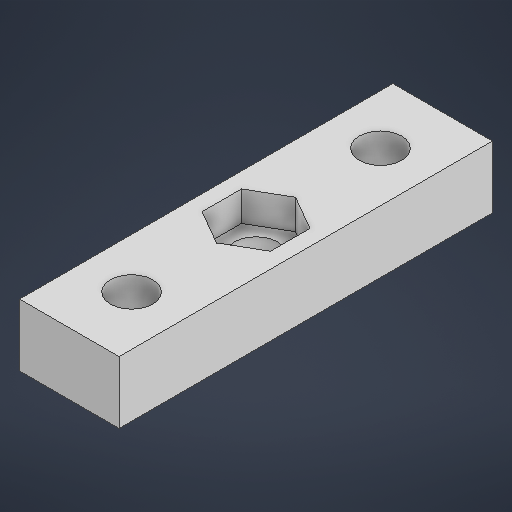
# Autodesk Inventor part: turning clip bottom
Saved by Autodesk Inventor 2025.2 (Build 292293000, 293)
## iProperties
Created: 2025-05-25
Part Number: turning clip bottom
Material: Generic
Document SubType Name: Modeling
Designer: klawy
Density: 1 g/cm^3
Appearance: Default
Author: klawy
Autodesk Inventor part; units mm, degrees
ref_plane "YZ Plane" through (0, 0, 0) normal (1, 0, 0) x (0, 1, 0)
ref_plane "XZ Plane" through (0, 0, 0) normal (0, 1, 0) x (-1, 0, 0)
ref_plane "XY Plane" through (0, 0, 0) normal (0, 0, 1) x (1, 0, 0)
sketch "Sketch1" plane through (0, 0, 0) normal (0, 1, 0) x (-1, 0, 0)
  line L0 (-4, -15) -> (4, -15)
  line L1 (4, -15) -> (4, 15)
  line L2 (4, 15) -> (-4, 15)
  line L3 (-4, 15) -> (-4, -15)
  line L4 (-4, -15) -> (4, 15) construction
  line L5 (4, -15) -> (-4, 15) construction
  circle A0 centre (0, 0) radius 1.75
  dimension "d0" = 8
  dimension "d1" = 30
  dimension "d2" = 3.5
  constraints: 12 end point, 2 midpoint, 2 parallel, 1 centre point, 1 coincident, 1 horizontal, 1 perpendicular
  measures "d0" distance of L1.end L2.end
  measures "d1" distance of L0.end L1.end
  measures "d2" diameter of A0
extrude "Extrusion1" add sketch "Sketch1" along normal blind 5
sketch "Sketch2" plane through (0, 5, 0) normal (0, 1, 0) x (1, 0, 0)
  circle A0 centre (0, 0) radius 1.75 projected
  circle A1 centre (0, 0) radius 2.75 construction
  line L0 (-2.75, 1.5877) -> (0, 3.1754)
  line L1 (0, 3.1754) -> (2.75, 1.5877)
  line L2 (2.75, 1.5877) -> (2.75, -1.5877)
  line L3 (2.75, -1.5877) -> (0, -3.1754)
  line L4 (0, -3.1754) -> (-2.75, -1.5877)
  line L5 (-2.75, -1.5877) -> (-2.75, 1.5877)
  point P0 (-2.75, 0)
  dimension "d5" = 5.5
  constraints: 12 end point, 2 coincident, 1 horizontal alignment, 1 midpoint, 1 vertical, 15 other
extrude "Extrusion2" cut sketch "Sketch2" against normal blind 2.4 contours A0 | L0 L1 L2 L3 L4 L5
sketch "Sketch3" plane through (0, 5, 0) normal (0, 1, 0) x (1, 0, 0)
  line L0 (-4, -15) -> (4, -15) projected
  line L1 (0, -15) -> (0, 15) construction
  line L2 (4, 15) -> (-4, 15) projected
  point P0 (0, 0)
  point P1 (0, -10)
  point P2 (0, 10)
  dimension "d8" = 5
  dimension "d9" = 5
  constraints: 2 end point, 2 midpoint, 2 point on line
  measures "d8" distance from line of L0 point (0, -10)
  measures "d9" distance from line of L2 point (0, 10)
hole "Hole1" at (0, 5, 10) at (0, 5, -10) direction (0, -1, 0) diameter 3.4 end through all clearance for "Countersunk Flat Head Screw ISO 2009/7046" size "M3" standard "ISO"
body "Solid1"
